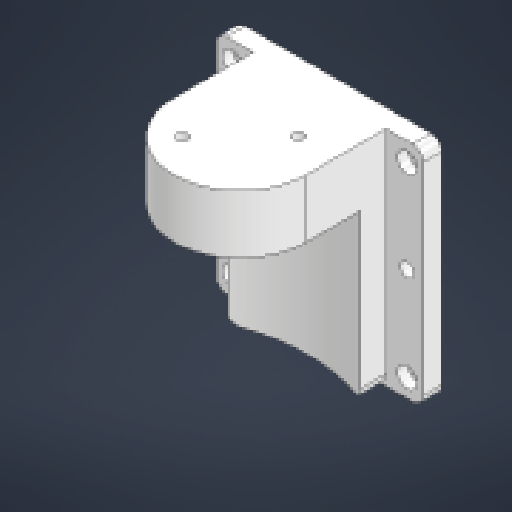
# Autodesk Inventor part: Dam1
Saved by Autodesk Inventor 2027 (Build 310192060, 192F)
## iProperties
Created: 2026-08-17
Part Number: Dam1
Material: PPS Plastic
Document SubType Name: Modeling
Designer: trtrn
Density: 1.637 g/cm^3
Appearance: Smooth - White
Author: trtrn
Autodesk Inventor part; units mm, degrees
ref_plane "YZ Plane" through (0, 0, 0) normal (1, 0, 0) x (0, 1, 0)
ref_plane "XZ Plane" through (0, 0, 0) normal (0, 1, 0) x (-1, 0, 0)
ref_plane "XY Plane" through (0, 0, 0) normal (0, 0, 1) x (1, 0, 0)
sketch "Sketch1" plane through (0, 0, 0) normal (0, 0, 1) x (1, 0, 0)
  line L0 (-39, 27.5) -> (39, 27.5)
  line L1 (39, 27.5) -> (39, -52.5)
  line L2 (39, -52.5) -> (-39, -52.5)
  line L3 (-39, -52.5) -> (-39, 27.5)
  line L4 (0, -52.5) -> (0, 27.5) construction
  point P0 (0, 0)
  dimension "d0" = 78
  dimension "d48" = 80
  dimension "d49" = 52.5
  constraints: 10 end point, 2 midpoint, 2 parallel, 1 horizontal, 1 perpendicular, 1 point on line
  measures "d0" distance of L1.end L2.end
  measures "d48" distance between parallel lines of L2 L0
  measures "d49" distance from line of L2 point (0, 0)
extrude "Extrusion1" add sketch "Sketch1" along normal blind 10
sketch "Sketch14" plane through (0, 0, 10) normal (0, 0, 1) x (1, 0, 0)
  line L0 (-25, 7.5) -> (25, 7.5)
  line L1 (25, 7.5) -> (25, 27.5)
  line L2 (25, 27.5) -> (-25, 27.5)
  line L3 (-25, 27.5) -> (-25, 7.5)
  line L4 (-25, 7.5) -> (25, 27.5) construction
  line L5 (25, 7.5) -> (-25, 27.5) construction
  line L6 (39, 27.5) -> (-39, 27.5) projected
  point P0 (0, 0)
  point P1 (0, 17.5)
  dimension "d50" = 50
  dimension "d51" = 20
  constraints: 12 end point, 2 midpoint, 2 parallel, 1 collinear, 1 horizontal, 1 perpendicular, 1 vertical alignment
  measures "d50" distance of L2.end L1.end
  measures "d51" distance of L1.end L0.end
extrude "Extrusion15" add sketch "Sketch14" along normal blind 30
sketch "Sketch15" plane through (-39, 27.5, 0) normal (0, 1, 0) x (1, 0, 0)
  line L0 (64, -40) -> (14, -40) projected
  circle A0 centre (39, -40) radius 25
  point P0 (39, 0)
  point P1 (64, -40)
  constraints: 1 midpoint, 3 other
extrude "Extrusion16" add sketch "Sketch15" against normal up to surface (20 mm away) contours A0 L0 picked at (37.9955, -48.2726)
sketch "Sketch17" plane through (-39, 27.5, 0) normal (0, 1, 0) x (1, 0, 0)
  circle A0 centre (39, -40) radius 19
  arc A1 (14, -40) -> (64, -40) centre (39, -40) ccw projected
  point P0 (39, 0)
  dimension "d62" = 38
  constraints: 1 centre point, 1 concentric
  measures "d62" diameter of A0
extrude "Extrusion17" cut sketch "Sketch17" against normal through all
extrude "Extrusion21" add sketch "Sketch17" against normal blind 15
sketch "Sketch22" plane through (0, 0, 10) normal (0, 0, 1) x (1, 0, 0)
  circle A0 centre (-33, 22.5) radius 1.65 construction
  circle A1 centre (-33, -12.5) radius 2.5 construction
  circle A2 centre (-33, -47.5) radius 1.65 construction
  circle A3 centre (33, -47.5) radius 1.65 construction
  circle A4 centre (33, -12.5) radius 2.5 projected
  circle A5 centre (33, 22.5) radius 1.65 projected
  point P0 (0, 0)
  constraints: 4 coincident
hole "Hole2" at (-33, 22.5, 10) at (-33, -47.5, 10) at (33, -47.5, 10) at (33, 22.5, 10) direction (0, 0, -1) diameter 4.3 end through all counterbore diameter 7.52 counterbore depth 4
sketch "Sketch23" plane through (0, 0, 10) normal (0, 0, 1) x (1, 0, 0)
  circle A0 centre (33, -12.5) radius 2.5 projected
  circle A1 centre (-33, -12.5) radius 2.5 construction
  point P0 (0, 0)
  constraints: 2 coincident
sketch "Sketch24" plane through (0, 0, 10) normal (0, 0, 1) x (1, 0, 0)
  point P0 (0, 0)
  point P1 (33, -12.5)
  point P2 (33, -12.5)
  point P3 (-33, -12.5)
  point P4 (-33, -12.5)
  point P5 (33, -12.5)
  constraints: 2 coincident
hole "Hole3" at (-33, -12.5, 10) at (33, -12.5, 10) direction (0, 0, -1) diameter 5.3 end through all
sketch "Sketch30" plane through (0, 12.5, 40) normal (0, -1, 0) x (1, 0, 0)
  line L0 (0.85, 1.55) -> (0.85, 16.5913)
  line L1 (16.1931, 1.05) -> (1.35, 1.05)
  line L2 (-0.85, 16.5913) -> (-0.85, 1.55)
  line L3 (-1.35, 1.05) -> (-16.1932, 1.05)
  line L4 (1.35, -1.05) -> (16.1931, -1.05)
  line L5 (0.85, -16.5913) -> (0.85, -1.55)
  line L6 (-16.1932, -1.05) -> (-1.35, -1.05)
  line L7 (-0.85, -1.55) -> (-0.85, -16.5913)
  point P0 (0, -40)
  point P1 (-10.85, 11.05)
  point P2 (10.85, -11.05)
  dimension "d123" = 10
  dimension "d124" = 10
  dimension "d125" = 10
  dimension "d126" = 10
  constraints: 16 end point, 4 horizontal, 4 vertical, 16 other
  measures "d123" distance from line of L2 point (-10.85, 11.05)
  measures "d124" distance from line of L3 point (-10.85, 11.05)
  measures "d125" distance from line of point (10.85, -11.05) L4
  measures "d126" distance from line of point (10.85, -11.05) L5
hole "Hole4" at (-10.85, 12.5, 51.05) at (10.85, 12.5, 28.95) direction (0, 1, 0) diameter 4.3 end through all
sketch "Sketch31" plane through (-25, 7.5, 10) normal (0, -1, 0) x (1, 0, 0)
  circle A0 centre (25, 30) radius 19 projected
  ellipse E0 centre (25, 30) end of major axis (66, 30) minor radius 25.625 (0, 9.6899) -> (50, 9.6899) ccw
  line L0 (0, 0) -> (0, 30) construction
  line L1 (50, 0) -> (50, 30) construction
  line L2 (0, 9.6899) -> (0, 0)
  line L3 (-14, 0) -> (64, 0) projected
  line L4 (50, 0) -> (50, 30) projected
  line L5 (50, 9.6899) -> (50, 0)
  line L6 (50, 0) -> (0, 0)
  point P0 (25, -10)
  dimension "d134" = 25.625
  dimension "d135" = 41
  constraints: 6 end point, 2 perpendicular, 2 point on line, 1 coincident, 1 collinear, 1 horizontal alignment, 4 other
extrude "Extrusion26" add sketch "Sketch31" along normal up to surface (60 mm away) contours E0 L4 L3 L2
sketch "Sketch34" plane through (0, 0, 0) normal (0, 0, -1) x (-1, 0, 0)
  line L0 (39, 27.5) -> (39, -52.5) projected
  line L1 (-39, 27.5) -> (39, 27.5) projected
  line L2 (-39, -52.5) -> (-39, 27.5) projected
  line L3 (39, -52.5) -> (-39, -52.5) projected
  point P0 (0, 0)
extrude "Extrusion28" cut sketch "Sketch34" against normal blind 3
move faces "Move1" translate (0, -2, 0) faces at (-8.3333, -52.5, 5.3333)
move faces "Move2" translate (0, 2, 0) faces at (-13.7614, 27.5, 26.2303)
fillet "Fillet2" radius 4 6 edges at (-39, 29.5, 6.5) (-39, -54.5, 6.5) (39, -54.5, 6.5) (39, 29.5, 6.5) (25, -54.5, 14.845) (-25, -54.5, 14.845)
body "Solid1"
